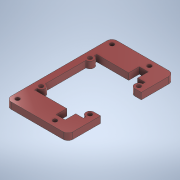
# Autodesk Inventor part: coupler
Saved by Autodesk Inventor 2021 (Build 250183000, 183)
## iProperties
Created: 2021-02-15
Part Number: coupler
Material: Generic
Document SubType Name: Modeling
Designer: lobato
Density: 1 g/cm^3
Appearance: Default
Author: lobato
Autodesk Inventor part; units mm, degrees
ref_plane "YZ Plane" through (0, 0, 0) normal (1, 0, 0) x (0, 1, 0)
ref_plane "XZ Plane" through (0, 0, 0) normal (0, 1, 0) x (-1, 0, 0)
ref_plane "XY Plane" through (0, 0, 0) normal (0, 0, 1) x (1, 0, 0)
sketch "Sketch1" plane through (0, 0, 0) normal (0, 1, 0) x (-1, 0, 0)
  line L0 (19, 32.5) -> (-11, 32.5)
  line L1 (-11, -32.5) -> (19, -32.5)
  line L2 (19, -32.5) -> (19, 32.5)
  line L3 (19, 32.5) -> (-19, -32.5) construction
  line L4 (-19, 32.5) -> (19, -32.5) construction
  line L5 (19, 19) -> (-19, 19) construction
  line L6 (-19, 19) -> (-19, -19) construction
  line L7 (-19, -19) -> (19, -19) construction
  line L8 (19, -19) -> (19, 19) construction
  line L9 (19, 19) -> (-19, -19) construction
  line L10 (-19, 19) -> (19, -19) construction
  line L11 (19, 32.5) -> (-11, 32.5) construction
  line L12 (-11, 32.5) -> (-11, -32.5) construction
  line L13 (-11, -32.5) -> (19, -32.5) construction
  line L14 (19, -32.5) -> (19, 32.5) construction
  line L15 (-21.9768, -11.3147) -> (-19, 12.5) construction
  line L16 (15.5, 29) -> (-7.5, 29) construction
  line L17 (-7.5, 29) -> (-7.5, -29) construction
  line L18 (-7.5, -29) -> (15.5, -29) construction
  line L19 (15.5, -29) -> (15.5, 29) construction
  line L20 (15, 15) -> (-15, 15) construction
  line L21 (-15, 15) -> (-15, -15) construction
  line L22 (-15, -15) -> (15, -15) construction
  line L23 (15, -15) -> (15, 15) construction
  line L24 (15, 15) -> (-15, -15) construction
  line L25 (-15, 15) -> (15, -15) construction
  circle A0 centre (15, 15) radius 1.25
  circle A1 centre (15, -15) radius 1.25
  circle A2 centre (-15, -15) radius 1.25
  circle A3 centre (-15, 15) radius 1.25
  circle A4 centre (-7.5, 29) radius 1.25
  circle A5 centre (15.5, 29) radius 1.25
  circle A6 centre (15.5, -29) radius 1.25
  circle A7 centre (-7.5, -29) radius 1.25
  circle A8 centre (0, 12) radius 2.5 construction
  circle A9 centre (0, -12) radius 2.5 construction
  line L26 (-4.75, 25.5) -> (-10.25, 25.5)
  line L27 (-10.25, 25.5) -> (-10.25, -25.5) construction
  line L28 (-10.25, -25.5) -> (-4.75, -25.5)
  line L29 (-4.75, -25.5) -> (-4.75, 25.5) construction
  line L30 (-4.75, 25.5) -> (-10.25, -25.5) construction
  line L31 (-10.25, 25.5) -> (-4.75, -25.5) construction
  line L32 (-11, 32.5) -> (-19, 32.5)
  line L33 (-19, 32.5) -> (-19, 19)
  line L34 (-19, -19) -> (-19, -32.5)
  line L35 (-19, -32.5) -> (-11, -32.5)
  arc A10 (-14.9077, -17.4983) -> (-15, -12.5) centre (-15, -15) ccw
  arc A11 (-15, 12.5) -> (-14.9077, 17.4983) centre (-15, 15) ccw
  line L36 (-15, 12.5) -> (-19, 12.5)
  line L37 (-19, 12.5) -> (-19, 19)
  line L38 (-15, -12.5) -> (-19, -12.5)
  line L39 (-19, -12.5) -> (-19, -19)
  line L40 (-14.9077, -17.4983) -> (-14.9077, -19)
  line L41 (-14.9077, 17.4983) -> (-14.9077, 19)
  arc A12 (15, 17.5) -> (15, 12.5) centre (15, 15) ccw
  line L42 (15, 12.5) -> (15, -12.5)
  line L43 (15, 17.5) -> (15, 19)
  line L44 (15, 19) -> (-4.75, 19)
  line L45 (-4.75, 19) -> (-4.75, 25.5)
  line L46 (-10.25, 25.5) -> (-10.25, 19)
  line L47 (-10.25, 19) -> (-14.9077, 19)
  line L48 (14.9077, -17.4983) -> (14.9077, -19)
  line L49 (14.9077, -19) -> (-4.75, -19)
  line L50 (-4.75, -19) -> (-4.75, -25.5)
  line L51 (-10.25, -25.5) -> (-10.25, -19)
  line L52 (-10.25, -19) -> (-14.9077, -19)
  arc A13 (15, -12.5) -> (14.9077, -17.4983) centre (15, -15) ccw
  point P0 (0, 0)
  point P1 (-7.5, 0)
  dimension "d0" = 38
  dimension "d2" = 38
  dimension "d3" = 38
  dimension "d4" = 30
  dimension "d8" = 65
  dimension "d9" = 23
  dimension "d10" = 58
  dimension "d11" = 3.5
  dimension "d13" = 3.5
  dimension "d14" = 2.5
  dimension "d15" = 2.5
  dimension "d16" = 2.5
  dimension "d17" = 2.5
  dimension "d18" = 2.5
  dimension "d19" = 2.5
  dimension "d20" = 2.5
  dimension "d21" = 2.5
  dimension "d22" = 5
  dimension "d23" = 5
  dimension "d24" = 7
  dimension "d25" = 7
  dimension "d31" = 5
  dimension "d32" = 5
  dimension "d33" = 4
  dimension "d34" = 5
  dimension "d36" = 5.5
  dimension "d37" = 51
  constraints: 106 end point, 22 point on line, 14 centre point, 12 coincident, 12 parallel, 11 perpendicular, 9 midpoint, 8 point on circle, 6 horizontal, 3 collinear, 1 tangent
  measures "d0" distance of L1.end L3.end
  measures "d2" distance of L6.end L7.end
  measures "d3" distance of L5.end L6.end
  measures "d4" distance of L1.start L13.end
  measures "d8" distance between parallel lines of L1 L0
  measures "d9" distance of L18.end L17.end
  measures "d10" distance of L17.end L16.end
  measures "d11" distance between parallel lines of L2 L19
  measures "d13" distance between parallel lines of L13 L18
  measures "d14" diameter of A0
  measures "d15" diameter of A1
  measures "d16" diameter of A2
  measures "d17" diameter of A3
  measures "d18" diameter of A4
  measures "d19" diameter of A5
  measures "d20" diameter of A6
  measures "d21" diameter of A7
  measures "d22" diameter of A8
  measures "d23" diameter of A9
  measures "d24" distance from line of L5 A8.centre
  measures "d25" distance from line of L7 A9.centre
  measures "d31" diameter of A10
  measures "d32" diameter of A11
  measures "d33" distance of L38.start L38.end
  measures "d34" diameter of A12
  measures "d36" distance of L27.end L28.end
  measures "d37" distance between parallel lines of L28 L26
extrude "Extrusion1" add sketch "Sketch1" along normal blind 4
fillet "Fillet1" radius 3 4 edges at (-19, 2, 32.5) (19, 2, 32.5) (19, 2, -32.5) (-19, 2, -32.5)
body "Solid1"
